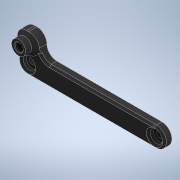
# Autodesk Inventor part: RodHolder_Back
Saved by Autodesk Inventor 2021 (Build 250183000, 183)
## iProperties
Created: 2020-07-16
Part Number: RodHolder_Back
Material: Generic
Document SubType Name: Modeling
Designer: CASE-SMALL2
Density: 1 g/cm^3
Appearance: Default
Author: CASE-SMALL2
## iProperties of the stored document _3DPrint.ipt
Created: 2020-07-21
Part Number: _3DPrint
Material: Generic
Document SubType Name: Modeling
Designer: CASE-SMALL2
Density: 1 g/cm^3
Appearance: Default
Author: CASE-SMALL2
Autodesk Inventor part; units mm, degrees
ref_plane "YZ Plane" through (0, 0, 0) normal (1, 0, 0) x (0, 1, 0)
ref_plane "XZ Plane" through (0, 0, 0) normal (0, 1, 0) x (-1, 0, 0)
ref_plane "XY Plane" through (0, 0, 0) normal (0, 0, 1) x (1, 0, 0)
sketch "Sketch1" plane through (0, 0, 0) normal (0, 0, 1) x (1, 0, 0)
  line L0 (-64, 0) -> (64, 0) construction
  line L1 (-64, -10) -> (64, -10)
  line L2 (64, 10) -> (-64, 10)
  arc A0 (-64, 10) -> (-64, -10) centre (-64, 0) ccw
  arc A1 (64, -10) -> (64, 10) centre (64, 0) ccw
  circle A2 centre (-64, 0) radius 3
  circle A3 centre (64, 0) radius 3
  point P0 (0, 0)
  dimension "d0" = 128
  dimension "d1" = 20
  dimension "d2" = 6
  dimension "d3" = 6
  constraints: 8 end point, 4 centre point, 4 point on circle, 4 tangent, 2 coincident, 1 horizontal, 1 midpoint, 1 parallel
  measures "d0" distance of L2.start L2.end
  measures "d1" distance between parallel lines of L1 L2
  measures "d2" diameter of A2
  measures "d3" diameter of A3
extrude "Extrusion1" add sketch "Sketch1" along normal blind 8
sketch "Sketch2" plane through (0, 0, 8) normal (0, 0, 1) x (1, 0, 0)
  circle A0 centre (-64, 0) radius 3 projected
  circle A1 centre (64, 0) radius 3 projected
  circle A2 centre (-64, 0) radius 6.25
  circle A3 centre (64, 0) radius 6.25
  point P0 (0, 0)
  dimension "d6" = 12.5
  dimension "d7" = 12.5
  constraints: 2 centre point, 2 coincident
  measures "d6" diameter of A2
  measures "d7" diameter of A3
ref_plane "Work Plane1" through (0, 0, 3) normal (0, 0, -1) x (-1, 0, 0)
extrude "Extrusion2" cut sketch "Sketch2" against normal up to surface (5 mm away)
chamfer "Chamfer1" distance 2 angle 45 2 edges at (-70.25, 0, 8) (57.75, 0, 8)
sketch "Sketch3" plane through (0, 0, 0) normal (0, 0, -1) x (-1, 0, 0)
  line L0 (52, 10) -> (52, 30)
  line L1 (52, 30) -> (74, 30)
  line L2 (74, 30) -> (74, 0)
  arc A0 (64, -10) -> (64, 10) centre (64, 0) ccw projected
  line L3 (-64, 10) -> (64, 10) projected
  point P0 (0, 0)
  dimension "d14" = 90
  dimension "d15" = 20
  dimension "d16" = 22
  constraints: 6 end point, 1 perpendicular, 1 point on circle, 1 point on line, 1 tangent, 1 vertical
  measures "d14" angle of L1 L2
  measures "d15" distance of L0.start L0.end
  measures "d16" distance of L0.end L1.end
extrude "Extrusion3" add sketch "Sketch3" against normal up to surface (8 mm away)
fillet "Fillet1" radius 10 3 edges at (-52, 10, 4) (-52, 30, 4) (-74, 30, 4)
sketch "Sketch4" plane through (0, 0, 8) normal (0, 0, 1) x (1, 0, 0)
  circle A0 centre (-63, 20) radius 4.15
  line L0 (-74, 0) -> (-74, 20) projected
  circle A1 centre (-64, 0) radius 3 projected
  circle A2 centre (-63, 20) radius 7.15
  point P0 (0, 0)
  dimension "d20" = 8.3
  dimension "d21" = 11
  dimension "d23" = 20
  dimension "d24" = 3
  constraints: 2 centre point, 1 coincident
  measures "d20" diameter of A0
  measures "d21" distance from line of L0 A0.centre
  measures "d23" vertical distance of A1.centre A0.centre
  measures "d24" radial gap between concentric circles of A2 A0
extrude "Extrusion4" add sketch "Sketch4" along normal blind 10 contours A2
chamfer "Chamfer2" distance 4 angle 45 1 edges at (-70.15, 20, 8)
chamfer "Chamfer3" distance 0.5 angle 45 1 edges at (-67.15, 20, 18)
chamfer "Chamfer4" distance 2 angle 45 6 edges at (11, 10, 8) (-48.6124, 12.4982, 8) (74, 0, 8) (0, -10, 8) (-71.0711, -7.0711, 8) (-74, 9.0886, 8)
chamfer "Chamfer5" distance 0.5 angle 45 10 edges at (11, 10, 0) (-52, 20, 0) (-49.0711, 12.9289, 0) (-54.9289, 27.0711, 0) (-63, 30, 0) (-71.0711, 27.0711, 0) (-74, 10.0001, 0) (-71.0711, -7.0711, 0) (0, -10, 0) (74, 0, 0)
equation "\"d3\" = d2"
equation "\"d7\" = d6"
body "Solid1"
